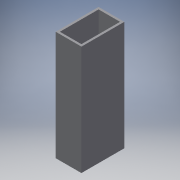
# Autodesk Inventor part: OUTERFrame Croner Opposite
Saved by Autodesk Inventor 2017 (Build 210142000, 142)
## iProperties
Created: 2019-01-17
Part Number: OUTERFrame Croner Opposite
Material: Generic
Document SubType Name: Modeling
Designer: S346795925
Density: 1 g/cm^3
Appearance: Default
Author: S346795925
Autodesk Inventor part; units mm, degrees
ref_plane "YZ Plane" through (0, 0, 0) normal (1, 0, 0) x (0, 1, 0)
ref_plane "XZ Plane" through (0, 0, 0) normal (0, 1, 0) x (-1, 0, 0)
ref_plane "XY Plane" through (0, 0, 0) normal (0, 0, 1) x (1, 0, 0)
sketch "Sketch1" plane through (0, 0, 0) normal (0, 1, 0) x (-1, 0, 0)
  line L0 (0, 0) -> (-38.1, 0)
  line L1 (-38.1, 0) -> (-38.1, -63.5)
  line L2 (-38.1, -63.5) -> (0, -63.5)
  line L3 (0, -63.5) -> (0, 0)
  line L4 (-3.175, -3.175) -> (-34.925, -3.175)
  line L5 (-34.925, -3.175) -> (-34.925, -60.325)
  line L6 (-34.925, -60.325) -> (-3.175, -60.325)
  line L7 (-3.175, -60.325) -> (-3.175, -3.175)
  dimension "d0" = 38.1
  dimension "d1" = 63.5
  dimension "d2" = 3.175
  constraints: 16 end point, 4 parallel, 2 perpendicular, 1 horizontal, 3 other
  measures "d0" distance of L2.end L1.end
  measures "d1" distance of L1.end L0.end
  measures "d2" distance between parallel lines of L3 L7
extrude "Extrusion1" add sketch "Sketch1" along normal blind 161.925
sketch "Sketch3" plane through (0, 0, -63.5) normal (-1, 0, 0) x (0, 0, 1)
  circle A0 centre (-68.6336, 53.0899) radius 53.4052
  circle A1 centre (-68.6336, 53.0899) radius 104.14
  point P0 (63.5, 0)
  dimension "d9" = 208.28
  constraints: 2 centre point, 1 coincident
  measures "d9" diameter of A1
extrude "Extrusion4" cut sketch "Sketch3" against normal blind 19.05 contours A0 | A1
body "Solid1"
